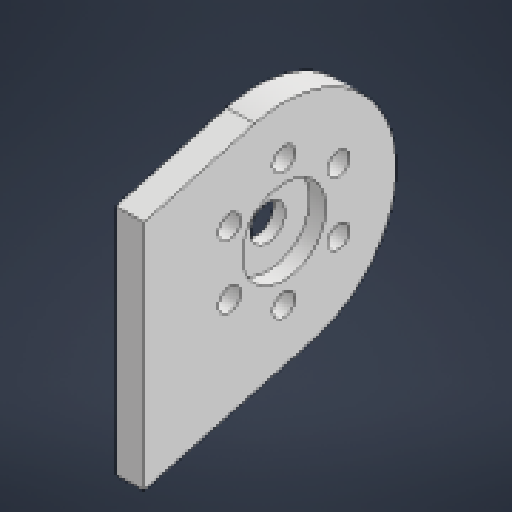
# Autodesk Inventor part: MotorMount
Saved by Autodesk Inventor 2024.2 (Build 282272000, 272)
## iProperties
Created: 2023-12-29
Part Number: MotorMount
Material: 一般
Document SubType Name: Modeling
Designer: Hanaoka
Density: 1 g/cm^3
Appearance: 既定
Author: Hanaoka
Autodesk Inventor part; units mm, degrees
ref_plane "YZ Plane" through (0, 0, 0) normal (1, 0, 0) x (0, 1, 0)
ref_plane "XZ Plane" through (0, 0, 0) normal (0, 1, 0) x (-1, 0, 0)
ref_plane "XY Plane" through (0, 0, 0) normal (0, 0, 1) x (1, 0, 0)
sketch "スケッチ1" plane through (0, 0, 0) normal (1, 0, 0) x (0, 1, 0)
  circle A0 centre (0, 0) radius 3
  circle A1 centre (0, 0) radius 4.5 construction
  circle A2 centre (4.5, 0) radius 0.8
  circle A3 centre (2.25, 3.8971) radius 0.8
  circle A4 centre (-2.25, 3.8971) radius 0.8
  circle A5 centre (-4.5, 0) radius 0.8
  circle A6 centre (-2.25, -3.8971) radius 0.8
  circle A7 centre (2.25, -3.8971) radius 0.8
  line L0 (-13.8471, 0) -> (13.0825, 0) projected
  line L1 (6.2329, 11) -> (-10, 11)
  line L2 (-10, 11) -> (-7.8852, -1.3502)
  circle A8 centre (0, 0) radius 1.25
  line L3 (0, 0) -> (-10, 0) construction
  line L4 (-10, 0) -> (-10, 11) construction
  arc A9 (-7.8852, -1.3502) -> (7.8852, 1.3502) centre (0, 0) ccw
  line L5 (6.2329, 11) -> (7.8852, 1.3502)
  point P0 (7.5963, 0)
  dimension "d1" = 9
  dimension "d0" = 6
  dimension "d2" = 1.6
  dimension "d5" = 360
  dimension "d8" = 2.5
  dimension "d13" = 8
  dimension "d14" = 10
  dimension "d15" = 11
  constraints: 10 end point, 9 centre point, 3 coincident, 2 horizontal, 2 point on circle, 2 point on line, 2 tangent, 1 horizontal alignment, 1 parallel, 1 vertical, 15 other
  measures "d0" diameter of A0
  measures "d2" diameter of A2
  measures "d8" diameter of A8
  measures "d13" radius of A9
  measures "d14" distance of L3.start L3.end
  measures "d15" distance of L1.end L3.end
extrude "押し出し1" add sketch "スケッチ1" against normal blind 2 contours L0 A8 A0 | L0 A2 A9 L2 A5 A0 | A0 L0 A8 | A0 L0 A5 L2 L1 L5 A9 A2
extrude "押し出し2" cut sketch "スケッチ1" against normal blind 1.15 contours L0 A8 A0 | A0 L0 A8
